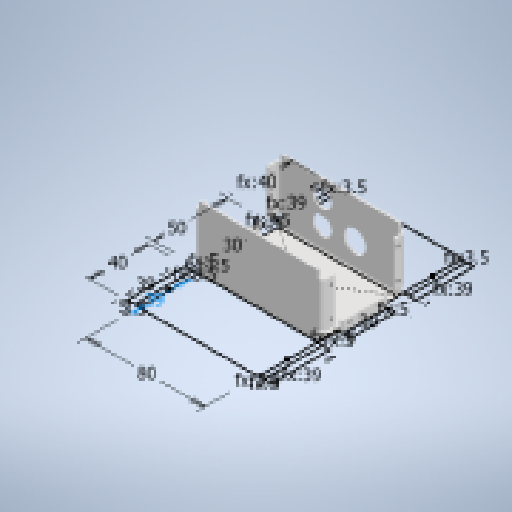
# Autodesk Inventor part: Bottom
Saved by Autodesk Inventor 2024 (Build 280153000, 153)
## iProperties
Created: 2025-10-28
Part Number: Bottom
Material: 일반
Document SubType Name: Sheet Metal
Designer: alexi
Density: 1 g/cm^3
Sheet Metal Rule: 기본값_mm
Appearance: 기본값
Author: alexi
Autodesk Inventor part; units mm, degrees
ref_plane "YZ Plane" through (0, 0, 0) normal (1, 0, 0) x (0, 1, 0)
ref_plane "XZ Plane" through (0, 0, 0) normal (0, 1, 0) x (-1, 0, 0)
ref_plane "XY Plane" through (0, 0, 0) normal (0, 0, 1) x (1, 0, 0)
sketch "Holes" plane through (0, 0, 0) normal (0, 0, 1) x (1, 0, 0)
  circle A0 centre (-13.7245, -10.9519) radius 4.4501 construction
  circle A1 centre (-13.7245, -26.9514) radius 4.0754 construction
  circle A2 centre (-35.7245, -25.0992) radius 0.9 construction
  point P0 (-21.0578, -21.0008)
sketch "PCB Holes" plane through (0, 0, 0) normal (0, 0, 1) x (1, 0, 0)
  circle A0 centre (-19.0196, -39.1634) radius 8.8876 construction
  circle A1 centre (2.9804, -41.0157) radius 7.94 construction
  circle A2 centre (2.9804, -25.0162) radius 7.94 construction
  line L0 (20.9804, -49.4134) -> (-39.0196, -49.4134) construction
  line L1 (20.9804, -50.0372) -> (-39.0196, -50.0372) construction
  line L2 (-39.0196, -50.0372) -> (-39.0196, -49.4134) construction
  line L3 (20.9804, -50.0372) -> (20.9804, -49.4134) construction
  point P0 (-7.4641, -44.8386)
sketch "스케치1" plane through (0, 0, 0) normal (0, 1, 0) x (-1, 0, 0)
  line L0 (40, -25) -> (-40, -25)
  line L1 (-40, -25) -> (-40, 25)
  line L2 (-40, 25) -> (40, 25)
  line L3 (40, 25) -> (40, -25)
  line L4 (40, -25) -> (-40, -25)
  line L5 (-40, -25) -> (-40, -28.5)
  line L6 (-40, -28.5) -> (40, -28.5)
  line L7 (40, -28.5) -> (40, -25)
  line L8 (40, 25) -> (-40, 25)
  line L9 (-40, 25) -> (-40, 28.5)
  line L10 (-40, 28.5) -> (40, 28.5)
  line L11 (40, 28.5) -> (40, 25)
  line L12 (40, 28.5) -> (-40, 28.5)
  line L13 (-40, 28.5) -> (-40, 68.5)
  line L14 (-40, 68.5) -> (40, 68.5)
  line L15 (40, 68.5) -> (40, 28.5)
  line L16 (40, -28.5) -> (-40, -28.5)
  line L17 (-40, -28.5) -> (-40, -68.5)
  line L18 (-40, -68.5) -> (40, -68.5)
  line L19 (40, -68.5) -> (40, -28.5)
  line L20 (40, 25) -> (-40, -25) construction
  line L21 (40, -25) -> (-40, 25) construction
  line L22 (40, 26.75) -> (-40, 26.75) construction
  line L23 (40, -26.75) -> (-40, -26.75) construction
  line L24 (40, -15) -> (43.5, -15)
  line L25 (43.5, -15) -> (43.5, 15)
  line L26 (43.5, 15) -> (40, 15)
  line L27 (40, 15) -> (40, -15)
  line L28 (-40, -15) -> (-43.5, -15)
  line L29 (-43.5, -15) -> (-43.5, 15)
  line L30 (-43.5, 15) -> (-40, 15)
  line L31 (-40, 15) -> (-40, -15)
  line L32 (43.5, -15) -> (48.5, -15)
  line L33 (48.5, -15) -> (48.5, 15)
  line L34 (48.5, 15) -> (43.5, 15)
  line L35 (43.5, 15) -> (43.5, -15)
  line L36 (-43.5, -15) -> (-48.5, -15)
  line L37 (-48.5, -15) -> (-48.5, 15)
  line L38 (-48.5, 15) -> (-43.5, 15)
  line L39 (-43.5, 15) -> (-43.5, -15)
  line L40 (40, -66) -> (43.5, -66)
  line L41 (43.5, -66) -> (43.5, -31)
  line L42 (43.5, -31) -> (40, -31)
  line L43 (40, -31) -> (40, -66)
  line L44 (-40, -66) -> (-43.5, -66)
  line L45 (-43.5, -66) -> (-43.5, -31)
  line L46 (-43.5, -31) -> (-40, -31)
  line L47 (-40, -31) -> (-40, -66)
  line L48 (40, 31) -> (43.5, 31)
  line L49 (43.5, 31) -> (43.5, 66)
  line L50 (43.5, 66) -> (40, 66)
  line L51 (40, 66) -> (40, 31)
  line L52 (43.5, 31) -> (48.5, 31)
  line L53 (48.5, 31) -> (48.5, 66)
  line L54 (48.5, 66) -> (43.5, 66)
  line L55 (43.5, 66) -> (43.5, 31)
  line L56 (-43.5, -66) -> (-48.5, -66)
  line L57 (-48.5, -66) -> (-48.5, -31)
  line L58 (-48.5, -31) -> (-43.5, -31)
  line L59 (-43.5, -31) -> (-43.5, -66)
  line L60 (43.5, -66) -> (48.5, -66)
  line L61 (48.5, -66) -> (48.5, -31)
  line L62 (48.5, -31) -> (43.5, -31)
  line L63 (43.5, -31) -> (43.5, -66)
  line L64 (-40, 31) -> (-43.5, 31)
  line L65 (-43.5, 31) -> (-43.5, 66)
  line L66 (-43.5, 66) -> (-40, 66)
  line L67 (-40, 66) -> (-40, 31)
  line L68 (-43.5, 31) -> (-48.5, 31)
  line L69 (-48.5, 31) -> (-48.5, 66)
  line L70 (-48.5, 66) -> (-43.5, 66)
  line L71 (-43.5, 66) -> (-43.5, 31)
  point P0 (0, 0)
  point P1 (0, 0)
  point P2 (40, 0)
  point P3 (-40, 0)
  point P4 (-40, 15)
  point P5 (40, 15)
  point P6 (40, -48.5)
  point P7 (-40, -48.5)
  point P8 (40, 48.5)
  point P9 (-40, 48.5)
  point P10 (-40, -31)
  point P11 (40, -31)
  point P12 (-40, 66)
  point P13 (40, 66)
  dimension "d0" = 50
  dimension "d1" = 80
  dimension "d2" = 3.5
  dimension "d3" = 3.5
  dimension "d4" = 40
  dimension "d5" = 40
  dimension "d19" = 30
  dimension "d20" = 30
  dimension "d21" = 3.5
  dimension "d22" = 3.5
  dimension "d23" = 5
  dimension "d24" = 5
  dimension "d37" = 3.5
  dimension "d38" = 3.5
  dimension "d40" = 3.5
  dimension "d41" = 5
  dimension "d43" = 5
  dimension "d44" = 5
  dimension "d45" = 3.5
  dimension "d46" = 5
  dimension "d47" = 35
  dimension "d48" = 35
  dimension "d49" = 35
  dimension "d50" = 35
  constraints: 144 end point, 34 parallel, 18 midpoint, 17 horizontal, 17 perpendicular, 10 point on line, 1 coincident
  measures "d0" distance of L2.end L0.start
  measures "d1" distance of L13.end L14.end
  measures "d2" distance of L10.end L2.end
  measures "d3" distance of L6.end L0.start
  measures "d4" distance of L14.end L10.end
  measures "d5" distance of L18.end L6.end
  measures "d19" distance of L24.end L25.end
  measures "d20" distance of L28.end L29.end
  measures "d21" distance of L25.end L26.end
  measures "d22" distance of L29.end L30.end
  measures "d23" distance of L25.end L33.end
  measures "d24" distance of L29.end L37.end
  measures "d37" distance of L40.start L40.end
  measures "d38" distance of L44.start L44.end
  measures "d40" distance of L49.end L50.end
  measures "d41" distance of L49.end L53.end
  measures "d43" distance of L41.end L61.end
  measures "d44" distance of L45.end L57.end
  measures "d45" distance of L65.end L66.end
  measures "d46" distance of L69.end L65.end
  measures "d47" distance of L52.end L53.end
  measures "d48" distance of L68.end L69.end
  measures "d49" distance of L60.end L61.end
  measures "d50" distance of L56.end L57.end
extrude "판1" add sketch "스케치1" against normal blind 1.5
fold "접기11" angle 90 bend radius 1.5 thickness 1.5 k factor 0.44 line from (43.5, 0, 31) to (43.5, 0, 66) line at bend end moving side (1, 0, 0) folds toward (0, 1, 0)
fold "접기12" angle 90 bend radius 1.5 thickness 1.5 k factor 0.44 line from (-43.5, 0, 31) to (-43.5, 0, 66) line at bend end moving side (-1, 0, 0) folds toward (0, 1, 0)
fold "접기13" angle 90 bend radius 1.5 thickness 1.5 k factor 0.44 line from (43.5, 0, -15) to (43.5, 0, 15) line at bend end moving side (1, 0, 0) folds toward (0, 1, 0)
fold "접기14" angle 90 bend radius 1.5 thickness 1.5 k factor 0.44 line from (-43.5, 0, -15) to (-43.5, 0, 15) line at bend end moving side (-1, 0, 0) folds toward (0, 1, 0)
fold "접기15" angle 90 bend radius 1.5 thickness 1.5 k factor 0.44 line from (43.5, 0, -31) to (43.5, 0, -66) line at bend end moving side (1, 0, 0) folds toward (0, 1, 0)
fold "접기16" angle 90 bend radius 1.5 thickness 1.5 k factor 0.44 line from (-43.5, 0, -66) to (-43.5, 0, -31) line at bend end moving side (-1, 0, 0) folds toward (0, 1, 0)
fold "접기17" angle 90 bend radius 1.5 thickness 1.5 k factor 0.44 line from (40, 0, 28.5) to (-40, 0, 28.5) line at bend end moving side (0, 0, 1) folds toward (0, 1, 0)
fold "접기18" angle 90 bend radius 1.5 thickness 1.5 k factor 0.44 line from (40, 0, -28.5) to (-40, 0, -28.5) line at bend end moving side (0, 0, -1) folds toward (0, 1, 0)
sketch "스케치3" plane through (-43.1071, 4, -20.1071) normal (-1, 0, 0) x (0, 0, 1)
  line L0 (45.2142, 0) -> (45.2142, 35) projected
  line L1 (40.2142, 35) -> (45.2142, 35) projected
  line L2 (40.2142, 0) -> (40.2142, 35) projected
  line L3 (45.2142, 0) -> (40.2142, 0) projected
  line L4 (-5, 35) -> (-5, 0) projected
  line L5 (0, 0) -> (-5, 0) projected
  line L6 (0, 35) -> (0, 0) projected
  line L7 (-5, 35) -> (0, 35) projected
  line L8 (5.1071, -2.5) -> (35.1071, -2.5) projected
  line L9 (35.1071, 2.5) -> (35.1071, -2.5) projected
  line L10 (5.1071, 2.5) -> (35.1071, 2.5) projected
  line L11 (5.1071, -2.5) -> (5.1071, 2.5) projected
  line L12 (-2.5, 35) -> (-2.5, 0) construction
  line L13 (42.7142, 35) -> (42.7142, 0) construction
  line L14 (5.1071, 0) -> (35.1071, 0) construction
  point P0 (20.1071, -4)
  point P1 (-2.5, 5)
  point P2 (-2.5, 30)
  point P3 (10.1071, 0)
  point P4 (30.1071, 0)
  point P5 (42.7142, 5)
  point P6 (42.7142, 30)
  dimension "d135" = 5
  dimension "d136" = 5
  dimension "d137" = 5
  dimension "d138" = 5
  dimension "d139" = 5
  dimension "d140" = 5
  constraints: 6 end point, 6 midpoint, 6 point on line
  measures "d135" distance from line of L5 point (-2.5, 5)
  measures "d136" distance from line of L7 point (-2.5, 30)
  measures "d137" distance from line of L11 point (10.107, 0)
  measures "d138" distance from line of L9 point (30.107, 0)
  measures "d139" distance from line of L3 point (42.714, 5)
  measures "d140" distance from line of L1 point (42.714, 30)
hole "구멍1" at (-43.1071, 9, -22.6071) at (-43.1071, 4, -10) at (-43.1071, 4, 10) at (-43.1071, 9, 22.6071) at (-43.1071, 34, 22.6071) at (-43.1071, 34, -22.6071) direction (1, 0, 0) diameter 2.459 depth 1.5 tip angle 118 thread size "M3x0.5" class "6H" standard "ANSI Metric M Profile"
sketch "스케치4" plane through (43.1071, 4, 20.1071) normal (1, 0, 0) x (0, 0, -1)
  line L0 (-5, 35) -> (-5, 0) projected
  line L1 (0, 0) -> (-5, 0) projected
  line L2 (0, 35) -> (0, 0) projected
  line L3 (-5, 35) -> (0, 35) projected
  line L4 (5.1071, -2.5) -> (35.1071, -2.5) projected
  line L5 (35.1071, 2.5) -> (35.1071, -2.5) projected
  line L6 (5.1071, 2.5) -> (35.1071, 2.5) projected
  line L7 (5.1071, -2.5) -> (5.1071, 2.5) projected
  line L8 (45.2142, 0) -> (45.2142, 35) projected
  line L9 (40.2142, 35) -> (45.2142, 35) projected
  line L10 (40.2142, 0) -> (40.2142, 35) projected
  line L11 (45.2142, 0) -> (40.2142, 0) projected
  line L12 (-2.5, 35) -> (-2.5, 0) construction
  line L13 (5.1071, -2.5) -> (5.1071, 2.5) projected
  line L14 (5.1071, 0) -> (35.1071, 0) construction
  line L15 (42.7142, 0) -> (42.7142, 35) construction
  point P0 (20.1071, -4)
  point P1 (-2.5, 30)
  point P2 (-2.5, 5)
  point P3 (10.1071, 0)
  point P4 (30.1071, 0)
  point P5 (42.7142, 30)
  point P6 (42.7142, 5)
  dimension "d148" = 5
  dimension "d149" = 5
  dimension "d150" = 5
  dimension "d151" = 5
  dimension "d152" = 5
  dimension "d153" = 5
  constraints: 6 end point, 6 midpoint, 6 point on line
  measures "d148" distance from line of point (-2.5, 30) L3
  measures "d149" distance from line of L1 point (-2.5, 5)
  measures "d150" distance from line of L7 point (10.107, 0)
  measures "d151" distance from line of L5 point (30.107, 0)
  measures "d152" distance from line of L11 point (42.714, 5)
  measures "d153" distance from line of L9 point (42.714, 30)
hole "구멍2" at (43.1071, 34, 22.6071) at (43.1071, 9, 22.6071) at (43.1071, 4, 10) at (43.1071, 4, -10) at (43.1071, 9, -22.6071) at (43.1071, 34, -22.6071) direction (-1, 0, 0) diameter 2.459 depth 1.5 tip angle 118 thread size "M3x0.5" class "6H" standard "ANSI Metric M Profile"
sketch "스케치6" plane through (40, 41.5, -28.1071) normal (0, 0, -1) x (-1, 0, 0)
  line L0 (40, -41.5) -> (40, -36.5) construction
  line L1 (0, -41.5) -> (80, -41.5) projected
  arc A0 (48.7829, -5.929) -> (55.2171, -5.929) centre (52, -11.479) ccw
  line L2 (48.7829, -5.929) -> (55.2171, -5.929)
  arc A1 (48.7829, -21.9285) -> (55.2171, -21.9285) centre (52, -27.4785) ccw
  line L3 (48.7829, -21.9285) -> (55.2171, -21.9285)
  circle A2 centre (30, -25.6263) radius 7.5
  circle A3 centre (30, -25.6263) radius 8.8876 construction
  circle A4 centre (52, -27.4785) radius 7.94 construction
  circle A5 centre (52, -11.479) radius 7.94 construction
  line L4 (70, -35.8763) -> (10, -35.8763) construction
  line L5 (70, -36.5) -> (10, -36.5) construction
  line L6 (10, -36.5) -> (10, -35.8763) construction
  line L7 (70, -36.5) -> (70, -35.8763) construction
  dimension "d161" = 5
  dimension "d162" = 6.415
  dimension "d163" = 5.55
  dimension "d164" = 6.415
  dimension "d165" = 5.55
  dimension "d166" = 15
  constraints: 6 end point, 4 point on circle, 3 centre point, 2 parallel, 1 horizontal, 1 perpendicular, 4 other
  measures "d161" distance of L0.start L0.end
  measures "d162" radius of A0
  measures "d164" radius of A1
  measures "d166" diameter of A2
extrude "돌출1" cut sketch "스케치6" against normal blind 10
equation "\"d2\" = d40"
equation "\"d3\" = d40"
equation "\"d5\" = d4"
equation "\"d21\" = d40"
equation "\"d22\" = d40"
equation "\"d23\" = d41"
equation "\"d24\" = d41"
equation "\"d37\" = d40"
equation "\"d38\" = d40"
equation "\"d43\" = d41"
equation "\"d44\" = d41"
equation "\"d45\" = d40"
equation "\"d46\" = d41"
equation "\"d48\" = d47"
equation "\"d49\" = d47"
equation "\"d50\" = d47"
equation "\"d87\" = BendReliefWidth"
equation "\"d88\" = BendReliefDepth"
equation "\"d89\" = MinimumRemnant"
equation "\"d90\" = TransitionRadius"
equation "\"d93\" = BendReliefWidth"
equation "\"d94\" = BendReliefDepth"
equation "\"d95\" = MinimumRemnant"
equation "\"d96\" = TransitionRadius"
equation "\"d99\" = BendReliefWidth"
equation "\"d100\" = BendReliefDepth"
equation "\"d101\" = MinimumRemnant"
equation "\"d102\" = TransitionRadius"
equation "\"d105\" = BendReliefWidth"
equation "\"d106\" = BendReliefDepth"
equation "\"d107\" = MinimumRemnant"
equation "\"d108\" = TransitionRadius"
equation "\"d111\" = BendReliefWidth"
equation "\"d112\" = BendReliefDepth"
equation "\"d113\" = MinimumRemnant"
equation "\"d114\" = TransitionRadius"
equation "\"d117\" = BendReliefWidth"
equation "\"d118\" = BendReliefDepth"
equation "\"d119\" = MinimumRemnant"
equation "\"d120\" = TransitionRadius"
equation "\"d123\" = BendReliefWidth"
equation "\"d124\" = BendReliefDepth"
equation "\"d125\" = MinimumRemnant"
equation "\"d126\" = TransitionRadius"
equation "\"d129\" = BendReliefWidth"
equation "\"d130\" = BendReliefDepth"
equation "\"d131\" = MinimumRemnant"
equation "\"d132\" = TransitionRadius"
equation "\"TransitionRadius\" = BendRadius"
equation "\"BendReliefWidth\" = 1.5"
equation "\"BendReliefDepth\" = 0.75"
equation "\"MinimumRemnant\" = 3"
equation "\"BendRadius\" = 1.5"
